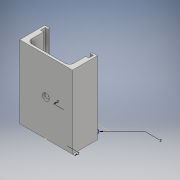
# Autodesk Inventor part: HB5_holder
Saved by Autodesk Inventor 2018 (Build 220112000, 112)
## iProperties
Created: 2018-04-27
Part Number: HB5_holder
Material: 一般
Document SubType Name: Modeling
Designer: izumi
Density: 1 g/cm^3
Appearance: 既定
Author: izumi
Autodesk Inventor part; units mm, degrees
ref_plane "YZ Plane" through (0, 0, 0) normal (1, 0, 0) x (0, 1, 0)
ref_plane "XZ Plane" through (0, 0, 0) normal (0, 1, 0) x (-1, 0, 0)
ref_plane "XY Plane" through (0, 0, 0) normal (0, 0, 1) x (1, 0, 0)
sketch "本体面" plane through (0, 0, 0) normal (0, 0, 1) x (1, 0, 0)
  line L0 (-11.6, 17) -> (11.6, 17)
  line L1 (11.6, 17) -> (11.6, 0)
  line L2 (11.6, 0) -> (-11.6, 0)
  line L3 (-11.6, 0) -> (-11.6, 17)
  point P0 (0, 0)
  point P1 (0, 0)
  dimension "d0" = 23.2
  dimension "d1" = 17
  constraints: 8 end point, 2 parallel, 1 coincident, 1 horizontal, 1 midpoint, 1 perpendicular
  measures "d0" distance of L1.end L2.end
  measures "d1" distance of L0.end L1.end
extrude "本体" add sketch "本体面" along normal blind 32
sketch "空洞面" plane through (0, 0, 32) normal (0, 0, 1) x (1, 0, 0)
  line L0 (-9.3, 11) -> (9.3, 11)
  line L1 (9.3, 11) -> (9.3, 3)
  line L2 (7.3, 1) -> (-7.3, 1)
  line L3 (-9.3, 3) -> (-9.3, 11)
  line L4 (11.6, 17) -> (-11.6, 17) projected
  arc A0 (-9.3, 3) -> (-7.3, 1) centre (-7.3, 3) ccw
  arc A1 (7.3, 1) -> (9.3, 3) centre (7.3, 3) ccw
  line L5 (-11.6, 0) -> (11.6, 0) projected
  point P0 (0, 0)
  point P1 (9.3, 1)
  point P2 (-9.3, 1)
  point P3 (0, 11)
  dimension "d4" = 18.6
  dimension "d6" = 2
  dimension "d31" = 1
  dimension "d32" = 10
  constraints: 8 end point, 4 point on circle, 4 point on line, 4 tangent, 2 centre point, 2 parallel, 1 equal radius, 1 horizontal, 1 midpoint, 1 perpendicular
  measures "d4" distance of point (9.3, 1) point (-9.3, 1)
  measures "d6" radius of A0
  measures "d31" distance between parallel lines of L5 L2
  measures "d32" distance between parallel lines of L2 L0
extrude "空洞" cut sketch "空洞面" against normal blind 32
sketch "左溝面" plane through (0, 0, 32) normal (0, 0, 1) x (1, 0, 0)
  line L0 (-10.6, 10.2) -> (-9.3, 10.2)
  line L1 (-9.3, 10.2) -> (-9.3, 8.2)
  line L2 (-9.3, 8.2) -> (-10.6, 8.2)
  line L3 (-10.6, 8.2) -> (-10.6, 10.2)
  line L4 (11.6, 17) -> (-11.6, 17) construction
  line L5 (-11.6, 17) -> (-11.6, 0) construction
  line L6 (-9.3, 3) -> (-9.3, 11) construction
  line L7 (-9.3, 11) -> (9.3, 11) construction
  point P0 (0, 0)
  point P1 (-9.3, 28)
  dimension "d10" = 2
  dimension "d28" = 1
  dimension "d33" = 0.8
  constraints: 8 end point, 2 parallel, 1 collinear, 1 horizontal, 1 perpendicular, 1 other
  measures "d10" distance of L0.end L1.end
  measures "d28" distance between parallel lines of L3 L5
  measures "d33" distance between parallel lines of L0 L7
extrude "左溝" cut sketch "左溝面" against normal blind 31
sketch "右溝面" plane through (0, 0, 32) normal (0, 0, 1) x (1, 0, 0)
  line L0 (9.3, 10.2) -> (10.6, 10.2)
  line L1 (10.6, 10.2) -> (10.6, 8.2)
  line L2 (10.6, 8.2) -> (9.3, 8.2)
  line L3 (9.3, 8.2) -> (9.3, 10.2)
  line L4 (11.6, 0) -> (11.6, 17) construction
  line L5 (9.3, 11) -> (9.3, 3) construction
  line L6 (-9.3, 11) -> (9.3, 11) construction
  point P0 (0, 0)
  dimension "d22" = 2
  dimension "d30" = 1
  dimension "d34" = 0.8
  constraints: 8 end point, 2 parallel, 1 collinear, 1 horizontal, 1 perpendicular
  measures "d22" distance of L2.end L0.start
  measures "d30" distance between parallel lines of L4 L1
  measures "d34" distance between parallel lines of L6 L0
extrude "右溝" cut sketch "右溝面" against normal blind 31
sketch "穴面" plane through (0, 0, 0) normal (0, 0, -1) x (-1, 0, 0)
  line L0 (-7.3, 15) -> (7.3, 15)
  line L1 (9.3, 13) -> (9.3, 4)
  line L2 (7.3, 2) -> (-7.3, 2)
  line L3 (-9.3, 4) -> (-9.3, 13)
  line L4 (11.6, 17) -> (-11.6, 17) construction
  line L5 (-11.6, 0) -> (11.6, 0) construction
  arc A0 (-7.3, 15) -> (-9.3, 13) centre (-7.3, 13) ccw
  arc A1 (9.3, 13) -> (7.3, 15) centre (7.3, 13) ccw
  arc A2 (-9.3, 4) -> (-7.3, 2) centre (-7.3, 4) ccw
  arc A3 (7.3, 2) -> (9.3, 4) centre (7.3, 4) ccw
  line L6 (9.3, 11) -> (9.3, 3) projected
  line L7 (-9.3, 3) -> (-9.3, 11) projected
  point P0 (0, 0)
  dimension "d41" = 2
  dimension "d44" = 2
  dimension "d45" = 2
  constraints: 8 end point, 8 point on circle, 8 tangent, 4 centre point, 3 equal radius, 2 collinear, 2 parallel, 1 horizontal, 1 perpendicular
  measures "d41" distance between parallel lines of L0 L4
  measures "d44" distance between parallel lines of L5 L2
  measures "d45" radius of A0
sketch "スケッチ11" plane through (0, 0, 32) normal (0, 0, 1) x (1, 0, 0)
  line L0 (-11.6, 17) -> (11.6, 17) projected
  line L1 (11.6, 17) -> (11.6, 0) projected
  line L2 (-11.6, 17) -> (11.6, 17)
  line L3 (11.6, 17) -> (11.6, 10.9937)
  line L4 (11.6, 10.9937) -> (-11.6, 10.9937)
  line L5 (-11.6, 10.9937) -> (-11.6, 17)
  point P0 (0, 0)
  constraints: 8 end point, 2 parallel, 1 horizontal, 1 perpendicular, 1 point on line
extrude "押し出し9" cut sketch "スケッチ11" along normal through all both and the other way through all
sketch "スケッチ12" plane through (-7.3, 1, 32) normal (0, 1, 0) x (1, 0, 0)
  line L0 (14.6, 0) -> (0, 0) projected
  line L1 (0, 0) -> (0, 32) projected
  line L2 (0, 0) -> (-2, 0) projected
  line L3 (14.6, 0) -> (14.6, 32) projected
  circle A0 centre (7.3, 16) radius 1.5
  point P0 (7.3, 32)
  dimension "d65" = 3
  constraints: 1 centre point
  measures "d65" diameter of A0
extrude "押し出し10" cut sketch "スケッチ12" against normal through all
